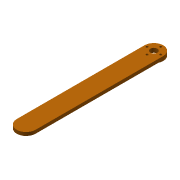
# Autodesk Inventor part: P_arm01_001
Saved by Autodesk Inventor 2016 (Build 200138000, 138)
## iProperties
Created: 2016-02-26
Part Number: P_arm01_001
Material: PC/ABS Plastic
Document SubType Name: Modeling
Designer: Mateusz
Density: 0.357273 g/cm^3
Appearance: Orange
Author: Mateusz
Autodesk Inventor part; units mm, degrees
ref_plane "YZ Plane" through (0, 0, 0) normal (1, 0, 0) x (0, 1, 0)
ref_plane "XZ Plane" through (0, 0, 0) normal (0, 1, 0) x (-1, 0, 0)
ref_plane "XY Plane" through (0, 0, 0) normal (0, 0, 1) x (1, 0, 0)
derived "skeleton.ipt"
sketch "Sketch1" plane through (0, 0, 0) normal (0, 0, 1) x (1, 0, 0)
  circle A0 centre (-0.9468, 0) radius 3.1 projected
  circle A1 centre (-0.9468, 8) radius 1.25 projected
  circle A2 centre (-8.9468, 0) radius 1.25 projected
  circle A3 centre (-0.9468, -8) radius 1.25 projected
  circle A4 centre (-6.4468, 0) radius 0.75 projected
  circle A5 centre (1.8032, 4.7631) radius 0.75 projected
  circle A6 centre (1.8032, -4.7631) radius 0.75 projected
  arc A7 (8.2786, 0.2472) -> (8.2786, -0.2472) centre (7.0532, 0) ccw projected
  line L0 (8.2786, 0.2472) -> (10.0505, 0.2472) projected
  arc A8 (10.0505, 0.2472) -> (-11.8865, 1.15) centre (-0.9468, 0) ccw projected
  line L1 (-11.8865, 1.15) -> (-11.5468, 1.15) projected
  line L2 (-11.5468, 1.15) -> (-11.5468, 0.85) projected
  line L3 (-11.5468, 0.85) -> (-11.9139, 0.85) projected
  arc A9 (-11.9139, 0.85) -> (-11.9139, -0.85) centre (-0.9468, 0) ccw projected
  line L4 (-11.9139, -0.85) -> (-11.5468, -0.85) projected
  line L5 (-11.5468, -0.85) -> (-11.5468, -1.15) projected
  line L6 (-11.5468, -1.15) -> (-11.8865, -1.15) projected
  arc A10 (-11.8865, -1.15) -> (10.0505, -0.2472) centre (-0.9468, 0) ccw projected
  line L7 (10.0505, -0.2472) -> (8.2786, -0.2472) projected
  circle A11 centre (-0.9468, 0) radius 11
  point P0 (0, 0)
  constraints: 1 centre point, 1 coincident, 1 concentric
extrude "Extrusion1" add sketch "Sketch1" along normal blind 1 contours A0 | A1 | A2 | A3 | A4 | A5 | A6 | L0 A11 L7 A7 | A7 L7 A10 L6 L5 L4 A9 L3 L2 L1 A8 L0 | L1 L2 L3 A11 | A11 L4 L5 L6
sketch "Sketch2" plane through (-0.9468, 0, 1) normal (0, 0, 1) x (1, 0, 0)
  circle A0 centre (0, 0) radius 11 projected
  circle A1 centre (0, 0) radius 11
  circle A2 centre (0, -60) radius 11
  circle A3 centre (0, 0) radius 11 projected
  line L0 (11, 0) -> (11, -60)
  line L1 (-11, -60) -> (-11, 0)
  point P0 (0.9468, 0)
  dimension "d3" = 60
  constraints: 6 point on circle, 4 end point, 4 tangent, 2 centre point, 2 equal radius, 1 coincident, 1 vertical
  measures "d3" distance of A2.centre A0.centre
extrude "Extrusion2" add sketch "Sketch2" along normal blind 4
sketch "Sketch3" plane through (-0.9468, 0, 5) normal (0, 0, 1) x (1, 0, 0)
  circle A0 centre (0, 0) radius 3.1 projected
  circle A1 centre (0, 8) radius 1.25 projected
  circle A2 centre (-8, 0) radius 1.25 projected
  circle A3 centre (0, -8) radius 1.25 projected
  circle A4 centre (-5.5, 0) radius 0.75 projected
  circle A5 centre (2.75, 4.7631) radius 0.75 projected
  circle A6 centre (2.75, -4.7631) radius 0.75 projected
  arc A7 (9.2253, 0.2472) -> (9.2253, -0.2472) centre (8, 0) ccw projected
  line L0 (9.2253, 0.2472) -> (10.9972, 0.2472) projected
  arc A8 (10.9972, 0.2472) -> (-10.9397, 1.15) centre (0, 0) ccw projected
  line L1 (-10.9397, 1.15) -> (-10.6, 1.15) projected
  line L2 (-10.6, 1.15) -> (-10.6, 0.85) projected
  line L3 (-10.6, 0.85) -> (-10.9671, 0.85) projected
  arc A9 (-10.9671, 0.85) -> (-10.9671, -0.85) centre (0, 0) ccw projected
  line L4 (-10.9671, -0.85) -> (-10.6, -0.85) projected
  line L5 (-10.6, -0.85) -> (-10.6, -1.15) projected
  line L6 (-10.6, -1.15) -> (-10.9397, -1.15) projected
  arc A10 (-10.9397, -1.15) -> (10.9972, -0.2472) centre (0, 0) ccw projected
  line L7 (10.9972, -0.2472) -> (9.2253, -0.2472) projected
  point P0 (0.9468, 0)
  constraints: 4 coincident
hole "Hole1" at (-8.9468, 0, 5) at (-0.9468, -8, 5) at (7.0532, 0, 5) at (-0.9468, 8, 5) direction (0, 0, -1) diameter 2.6 end through all
sketch "Sketch4" plane through (-0.9468, 0, 5) normal (0, 0, 1) x (1, 0, 0)
  circle A0 centre (0, 0) radius 3.1 projected
  circle A1 centre (0, 0) radius 4.1
  point P0 (0.9468, 0)
  dimension "d13" = 1
  constraints: 1 centre point
  measures "d13" radial gap between concentric circles of A0 A1
extrude "Extrusion3" cut sketch "Sketch4" against normal through all contours A0 | A1
equation "\"d3\" = arm_length"
equation "\"arm_length\" = 60"
body "Solid1"
